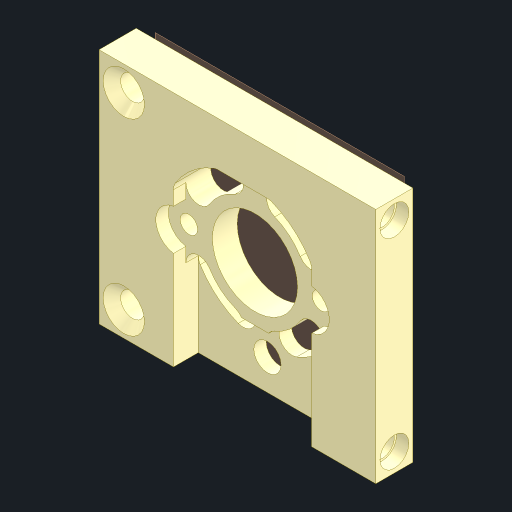
# Autodesk Inventor part: right_motor_front_mount
Saved by Autodesk Inventor 2023 (Build 270158000, 158)
## iProperties
Created: 2024-04-27
Part Number: right_motor_front_mount
Material: Nylon 6/6
Document SubType Name: Modeling
Designer: szymo
Density: 1.13 g/cm^3
Appearance: Nylon 6
Author: szymo
Autodesk Inventor part; units mm, degrees
ref_plane "YZ Plane" through (0, 0, 0) normal (1, 0, 0) x (0, 1, 0)
ref_plane "XZ Plane" through (0, 0, 0) normal (0, 1, 0) x (-1, 0, 0)
ref_plane "XY Plane" through (0, 0, 0) normal (0, 0, 1) x (1, 0, 0)
ref_plane "Work Plane1" through (0, 0, 0) normal (0, 0, 1) x (1, 0, 0)
sketch "Sketch1" plane through (0, 0, 0) normal (0, 0, 1) x (1, 0, 0)
  arc A0 (5.9062, 3.651) -> (7.7035, 4.7619) centre (6.8048, 4.2064) ccw projected
  arc A1 (5.9062, 3.651) -> (2.5768, 6.4477) centre (0, 0) ccw projected
  arc A2 (3.3608, 8.4097) -> (2.5768, 6.4477) centre (2.9688, 7.4287) ccw projected
  arc A3 (7.7035, 4.7619) -> (3.3608, 8.4097) centre (0, 0) ccw projected
  arc A4 (2.5768, -6.4477) -> (3.3608, -8.4097) centre (2.9688, -7.4287) ccw projected
  arc A5 (2.5768, -6.4477) -> (5.9062, -3.651) centre (0, 0) ccw projected
  arc A6 (7.7035, -4.7619) -> (5.9062, -3.651) centre (6.8048, -4.2064) ccw projected
  arc A7 (3.3608, -8.4097) -> (7.7035, -4.7619) centre (0, 0) ccw projected
  arc A8 (-2.5553, 6.4563) -> (-3.3328, 8.4209) centre (-2.9441, 7.4386) ccw projected
  arc A9 (-2.5553, 6.4563) -> (-5.9062, 3.651) centre (0, 0) ccw projected
  arc A10 (-7.7035, 4.7619) -> (-5.9062, 3.651) centre (-6.8048, 4.2064) ccw projected
  arc A11 (-3.3328, 8.4209) -> (-7.7035, 4.7619) centre (0, 0) ccw projected
  arc A12 (-5.9062, -3.651) -> (-7.7035, -4.7619) centre (-6.8048, -4.2064) ccw projected
  arc A13 (-5.9062, -3.651) -> (-2.5553, -6.4563) centre (0, 0) ccw projected
  arc A14 (-3.3328, -8.4209) -> (-2.5553, -6.4563) centre (-2.9441, -7.4386) ccw projected
  arc A15 (-7.7035, -4.7619) -> (-3.3328, -8.4209) centre (0, 0) ccw projected
  circle A16 centre (0.0124, -10.65) radius 1.15 projected
  circle A17 centre (8, 0) radius 1.0564 projected
  circle A18 centre (-8, 0) radius 1.0564 projected
  circle A19 centre (0, 0) radius 5 projected
  circle A20 centre (0, 0) radius 13.7 projected
  line L0 (0, 14.375) -> (-17.375, 14.375) projected
  line L1 (-17.375, 14.375) -> (-17.375, -14.375) projected
  line L2 (-17.375, -14.375) -> (0, -14.375) projected
  circle A21 centre (0, 0) radius 5.15
  arc A22 (5.4809, 3.3881) -> (8.1288, 5.0248) centre (6.8048, 4.2064) ccw
  arc A23 (5.4809, 3.3881) -> (2.3912, 5.9835) centre (0, 0) ccw
  arc A24 (3.5464, 8.874) -> (2.3912, 5.9835) centre (2.9688, 7.4287) ccw
  arc A25 (8.1288, 5.0248) -> (3.5464, 8.874) centre (0, 0) ccw
  arc A26 (8.1288, -5.0248) -> (5.4809, -3.3881) centre (6.8048, -4.2064) ccw
  arc A27 (2.3912, -5.9835) -> (5.4809, -3.3881) centre (0, 0) ccw
  arc A28 (2.3912, -5.9835) -> (3.5464, -8.874) centre (2.9688, -7.4287) ccw
  arc A29 (3.5464, -8.874) -> (8.1288, -5.0248) centre (0, 0) ccw
  circle A30 centre (0.0124, -10.65) radius 1.65
  arc A31 (-5.4809, -3.3881) -> (-2.3713, -5.9914) centre (0, 0) ccw
  arc A32 (-5.4809, -3.3881) -> (-8.1288, -5.0248) centre (-6.8048, -4.2064) ccw
  arc A33 (-8.1288, -5.0248) -> (-3.5168, -8.8858) centre (0, 0) ccw
  arc A34 (-3.5168, -8.8858) -> (-2.3713, -5.9914) centre (-2.9441, -7.4386) ccw
  arc A35 (-2.3713, 5.9914) -> (-5.4809, 3.3881) centre (0, 0) ccw
  arc A36 (-2.3713, 5.9914) -> (-3.5168, 8.8858) centre (-2.9441, 7.4386) ccw
  arc A37 (-3.5168, 8.8858) -> (-8.1288, 5.0248) centre (0, 0) ccw
  arc A38 (-8.1288, 5.0248) -> (-5.4809, 3.3881) centre (-6.8048, 4.2064) ccw
  circle A39 centre (-14.375, -11.375) radius 1.75 projected
  circle A40 centre (-14.375, 11.375) radius 1.75 projected
  arc A41 (0, 13.7) -> (0, -13.7) centre (0, 0) ccw projected
  line L3 (0, -14.375) -> (0, -13.7) projected
  line L4 (0, 13.7) -> (0, 14.375) projected
  line L5 (16.125, 8.6145) -> (16.125, -8.7895) projected
  line L6 (0, -14.375) -> (16.125, -14.375)
  line L7 (16.125, -14.375) -> (16.125, 14.375)
  line L8 (16.125, 14.375) -> (0, 14.375)
  line L9 (0, 14.375) -> (0, -14.375)
  point P0 (0, 0)
  dimension "d0" = 0.15
  dimension "d1" = 0.5
  dimension "d2" = 0.5
  dimension "d3" = 0.5
  dimension "d4" = 0.5
  dimension "d5" = 0.5
  constraints: 32 point on circle, 18 centre point, 8 end point, 2 parallel, 1 horizontal, 1 perpendicular, 12 other
  measures "d0" radial gap between concentric circles of A19 A21
  measures "d1" radial gap between concentric circles of A0 A22
  measures "d2" radial gap between concentric circles of A7 A29
  measures "d3" radial gap between concentric circles of A16 A30
  measures "d4" radial gap between concentric circles of A13 A31
  measures "d5" radial gap between concentric circles of A9 A35
extrude "Extrusion1" add sketch "Sketch1" along normal blind 1.5 contours L9 A21 A20 A30 | A30 L9 A20 A21 | L3 L2 L1 L0 L4 A20 | A20 L4 L8 L7 L5 L6 L3 | A39 | A40
sketch "Sketch2" plane through (0, 0, 1.5) normal (0, 0, 1) x (1, 0, 0)
  line L0 (-17.375, 14.375) -> (-17.375, -14.375) projected
  line L1 (-17.375, -14.375) -> (16.125, -14.375) projected
  line L2 (16.125, -14.375) -> (16.125, 14.375) projected
  line L3 (16.125, 14.375) -> (-17.375, 14.375) projected
  circle A0 centre (8, 0) radius 1.0564 projected
  circle A1 centre (-8, 0) radius 1.0564 projected
  circle A2 centre (0, 0) radius 5.15 projected
  arc A3 (5.4809, 3.3881) -> (2.3912, 5.9835) centre (0, 0) ccw projected
  arc A4 (3.5464, 8.874) -> (2.3912, 5.9835) centre (2.9688, 7.4287) ccw projected
  arc A5 (8.1288, 5.0248) -> (3.5464, 8.874) centre (0, 0) ccw projected
  arc A6 (5.4809, 3.3881) -> (8.1288, 5.0248) centre (6.8048, 4.2064) ccw projected
  arc A7 (2.3912, -5.9835) -> (5.4809, -3.3881) centre (0, 0) ccw projected
  arc A8 (8.1288, -5.0248) -> (5.4809, -3.3881) centre (6.8048, -4.2064) ccw projected
  arc A9 (3.5464, -8.874) -> (8.1288, -5.0248) centre (0, 0) ccw projected
  arc A10 (2.3912, -5.9835) -> (3.5464, -8.874) centre (2.9688, -7.4287) ccw projected
  circle A11 centre (0.0124, -10.65) radius 1.65 projected
  arc A12 (-5.4809, -3.3881) -> (-8.1288, -5.0248) centre (-6.8048, -4.2064) ccw projected
  arc A13 (-5.4809, -3.3881) -> (-2.3713, -5.9914) centre (0, 0) ccw projected
  arc A14 (-3.5168, -8.8858) -> (-2.3713, -5.9914) centre (-2.9441, -7.4386) ccw projected
  arc A15 (-8.1288, -5.0248) -> (-3.5168, -8.8858) centre (0, 0) ccw projected
  arc A16 (-2.3713, 5.9914) -> (-3.5168, 8.8858) centre (-2.9441, 7.4386) ccw projected
  arc A17 (-2.3713, 5.9914) -> (-5.4809, 3.3881) centre (0, 0) ccw projected
  arc A18 (-8.1288, 5.0248) -> (-5.4809, 3.3881) centre (-6.8048, 4.2064) ccw projected
  arc A19 (-3.5168, 8.8858) -> (-8.1288, 5.0248) centre (0, 0) ccw projected
  arc A20 (8.1288, -5.0248) -> (5.4809, -3.3881) centre (6.8048, -4.2064) ccw projected
  line L4 (8.3613, -4.2064) -> (8.3613, -14.375)
  line L5 (-17.375, -14.375) -> (16.125, -14.375) projected
  arc A21 (-5.4809, -3.3881) -> (-8.1288, -5.0248) centre (-6.8048, -4.2064) ccw projected
  line L6 (-8.3613, -4.2064) -> (-8.3613, -14.375)
  arc A22 (2.3912, -5.9835) -> (3.5464, -8.874) centre (2.9688, -7.4287) ccw projected
  line L7 (1.6624, -6.5827) -> (-1.6441, -6.5827)
  arc A23 (-3.5168, -8.8858) -> (-2.3713, -5.9914) centre (-2.9441, -7.4386) ccw projected
  point P0 (0, 0)
  constraints: 6 end point, 4 point on circle, 3 tangent, 2 perpendicular, 2 point on line, 1 horizontal
extrude "Extrusion2" add sketch "Sketch2" along normal blind 1.5 contours L3 L2 L1 L4 A8 A7 A10 L7 A14 A13 A12 L6 L0
sketch "Sketch3" plane through (0, 0, 3) normal (0, 0, 1) x (1, 0, 0)
  circle A0 centre (0, 0) radius 6.75 projected
  line L0 (-17.375, -14.375) -> (-8.3613, -14.375) projected
  line L1 (-8.3613, -14.375) -> (-8.3613, -4.2064) projected
  arc A1 (-5.4809, -3.3881) -> (-8.3613, -4.2064) centre (-6.8048, -4.2064) ccw projected
  arc A2 (-5.4809, -3.3881) -> (-2.3713, -5.9914) centre (0, 0) ccw projected
  arc A3 (-1.6441, -6.5827) -> (-2.3713, -5.9914) centre (-2.9441, -7.4386) ccw projected
  line L2 (-1.6441, -6.5827) -> (1.6624, -6.5827) projected
  arc A4 (2.3912, -5.9835) -> (1.6624, -6.5827) centre (2.9688, -7.4287) ccw projected
  arc A5 (2.3912, -5.9835) -> (5.4809, -3.3881) centre (0, 0) ccw projected
  arc A6 (8.3613, -4.2064) -> (5.4809, -3.3881) centre (6.8048, -4.2064) ccw projected
  line L3 (8.3613, -4.2064) -> (8.3613, -14.375) projected
  line L4 (8.3613, -14.375) -> (16.125, -14.375) projected
  line L5 (16.125, -14.375) -> (16.125, 14.375) projected
  line L6 (16.125, 14.375) -> (-17.375, 14.375) projected
  line L7 (-17.375, 14.375) -> (-17.375, -14.375) projected
  circle A7 centre (8, 0) radius 1.0564 projected
  circle A8 centre (-8, 0) radius 1.0564 projected
  arc A9 (-2.3713, 5.9914) -> (-5.4809, 3.3881) centre (0, 0) ccw projected
  arc A10 (-8.1288, 5.0248) -> (-5.4809, 3.3881) centre (-6.8048, 4.2064) ccw projected
  arc A11 (-3.5168, 8.8858) -> (-8.1288, 5.0248) centre (0, 0) ccw projected
  arc A12 (-2.3713, 5.9914) -> (-3.5168, 8.8858) centre (-2.9441, 7.4386) ccw projected
  arc A13 (5.4809, 3.3881) -> (8.1288, 5.0248) centre (6.8048, 4.2064) ccw projected
  arc A14 (5.4809, 3.3881) -> (2.3912, 5.9835) centre (0, 0) ccw projected
  arc A15 (3.5464, 8.874) -> (2.3912, 5.9835) centre (2.9688, 7.4287) ccw projected
  arc A16 (8.1288, 5.0248) -> (3.5464, 8.874) centre (0, 0) ccw projected
  circle A17 centre (0, 0) radius 5.15 projected
  circle A18 centre (8, 0) radius 2.5
  circle A19 centre (-8, 0) radius 2.5
  line L8 (2.9688, 8.9852) -> (-2.9441, 8.9852)
  line L9 (2.9688, 8.9852) -> (8.8817, 8.9852) construction
  arc A20 (-8.1288, 5.0248) -> (-5.4809, 3.3881) centre (-6.8048, 4.2064) ccw projected
  line L10 (-8.3613, 4.2064) -> (-8.3613, -4.2064)
  arc A21 (-5.4809, -3.3881) -> (-8.1288, -5.0248) centre (-6.8048, -4.2064) ccw projected
  arc A22 (5.4809, 3.3881) -> (8.1288, 5.0248) centre (6.8048, 4.2064) ccw projected
  line L11 (8.3613, 4.2064) -> (8.3613, -4.2064)
  point P0 (0, 0)
  point P1 (-8.3613, -2.4738)
  point P2 (-8.3613, 2.4738)
  point P3 (-2.7693, 8.9852)
  point P4 (8.3613, 2.4738)
  point P5 (8.3613, -2.4738)
  dimension "d10" = 5
  dimension "d11" = 5
  dimension "d12" = 180
  constraints: 8 end point, 3 point on circle, 3 tangent, 2 centre point, 2 coincident, 1 collinear, 1 horizontal, 1 parallel, 1 point on line
  measures "d10" diameter of A18
  measures "d11" diameter of A19
  measures "d12" angle of L8 L9
extrude "Extrusion3" add sketch "Sketch3" along normal blind 1.5 contours L11 A13 A16 A15 L8 A12 A11 A10 L10 A19 L1 L0 L7 L6 L5 L4 L3 A18
sketch "Sketch4" plane through (0, 0, 4.5) normal (0, 0, 1) x (1, 0, 0)
  line L0 (16.125, -14.375) -> (16.125, 14.375) projected
  line L1 (-17.375, -14.375) -> (16.125, -14.375) projected
  line L2 (16.125, 14.375) -> (12.625, 14.375)
  line L3 (12.625, -14.375) -> (16.125, -14.375)
  line L4 (16.125, -14.375) -> (16.125, 14.375)
  circle A0 centre (13.125, 11.375) radius 3
  circle A1 centre (13.125, -11.375) radius 3
  circle A2 centre (-14.375, -11.375) radius 3
  circle A3 centre (-14.375, 11.375) radius 3
  line L5 (-8.3613, -14.375) -> (-8.3613, -2.4738) projected
  arc A4 (-8.3613, 2.4738) -> (-8.3613, -2.4738) centre (-8, 0) ccw projected
  line L6 (-8.3613, 2.4738) -> (-8.3613, 4.2064) projected
  arc A5 (-8.1288, 5.0248) -> (-8.3613, 4.2064) centre (-6.8048, 4.2064) ccw projected
  arc A6 (-3.5168, 8.8858) -> (-8.1288, 5.0248) centre (0, 0) ccw projected
  arc A7 (-2.7693, 8.9852) -> (-3.5168, 8.8858) centre (-2.9441, 7.4386) ccw projected
  line L7 (-2.7693, 8.9852) -> (2.9688, 8.9852) projected
  arc A8 (3.5464, 8.874) -> (2.9688, 8.9852) centre (2.9688, 7.4287) ccw projected
  arc A9 (8.1288, 5.0248) -> (3.5464, 8.874) centre (0, 0) ccw projected
  arc A10 (8.3613, 4.2064) -> (8.1288, 5.0248) centre (6.8048, 4.2064) ccw projected
  line L8 (8.3613, 4.2064) -> (8.3613, 2.4738) projected
  arc A11 (8.3613, -2.4738) -> (8.3613, 2.4738) centre (8, 0) ccw projected
  line L9 (8.3613, -2.4738) -> (8.3613, -14.375) projected
  line L10 (8.3613, -14.375) -> (16.125, -14.375) projected
  line L11 (16.125, -14.375) -> (16.125, 14.375) projected
  line L12 (16.125, 14.375) -> (-17.375, 14.375) projected
  line L13 (-17.375, 14.375) -> (-17.375, -14.375) projected
  line L14 (-17.375, -14.375) -> (-8.3613, -14.375) projected
  point P0 (0, 0)
  dimension "d16" = 6
  dimension "d17" = 6
  dimension "d18" = 6
  dimension "d19" = 6
  constraints: 8 tangent, 6 end point, 4 centre point, 1 horizontal, 1 parallel, 1 point on line
  measures "d16" diameter of A0
  measures "d17" diameter of A1
  measures "d18" diameter of A2
  measures "d19" diameter of A3
hole "Hole1" at (-14.375, -11.375, 4.5) at (-14.375, 11.375, 4.5) direction (0, 0, -1) diameter 2.9 end through all countersink diameter 5 countersink angle 90 clearance for "Countersunk Flat Head Screw ISO 2009/7046" size "M2.5" standard "ISO"
sketch "Sketch6" plane through (16.125, -14.375, 0) normal (1, 0, 0) x (0, 0, -1)
  line L0 (0, 0) -> (0, 28.75) projected
  line L1 (0, 28.75) -> (-4.5, 28.75) projected
  line L2 (-4.5, 0) -> (-4.5, 28.75) projected
  line L3 (0, 0) -> (-4.5, 0) projected
  line L4 (0, 28.75) -> (-4.5, 28.75)
  line L5 (-4.5, 28.75) -> (-4.5, 24.25)
  line L6 (-4.5, 24.25) -> (0, 24.25)
  line L7 (0, 24.25) -> (0, 28.75)
  line L8 (0, 0) -> (-4.5, 0)
  line L9 (-4.5, 0) -> (-4.5, 4.5)
  line L10 (-4.5, 4.5) -> (0, 4.5)
  line L11 (0, 4.5) -> (0, 0)
  line L12 (-4.5, 24.25) -> (0, 28.75)
  line L13 (-4.5, 28.75) -> (0, 24.25)
  line L14 (0, 0) -> (-4.5, 0) projected
  line L15 (0, 4.5) -> (-4.5, 0)
  line L16 (0, 0) -> (-4.5, 4.5)
  point P0 (0, 14.375)
  point P1 (-2.25, 26.5)
  point P2 (-2.25, 2.25)
  dimension "d34" = 4.5
  dimension "d35" = 4.5
  dimension "d36" = 4.5
  dimension "d37" = 4.5
  constraints: 24 end point, 4 parallel, 3 perpendicular, 2 horizontal, 2 midpoint, 1 point on line
  measures "d34" distance of L6.end L5.end
  measures "d35" distance of L5.end L4.end
  measures "d36" distance of L9.end L10.end
  measures "d37" distance of L8.end L9.end
hole "Hole3" at (16.125, 12.125, 2.25) at (16.125, -12.125, 2.25) direction (-1, 0, 0) diameter 3 depth 3.5 counterbore diameter 3.5 counterbore depth 1.5
body "Solid1"
